OSD60-0_v9 (Autodesk Fusion 360 design; units mm, degrees)
Autodesk Fusion 360 part; units mm, degrees
sketch "Sketch1" plane through (0, 0, 0) normal (0, 0, 1) x (1, 0, 0)
  line L0 (6.985, 0.6858) -> (6.985, 4.1021)
  line L1 (6.223, 4.6101) -> (0, 4.6101)
  line L2 (0, 4.6101) -> (0, 0)
  line L3 (0, 0) -> (7.6581, 0)
  line L4 (7.6581, 0) -> (7.6581, 0.6858)
  line L5 (7.6581, 0.6858) -> (0, 0.6858)
  line L6 (0, 0.6858) -> (0, 0)
  line L7 (6.985, 4.1021) -> (6.223, 4.6101)
  point P0 (6.985, 4.6101)
  dimension "d2" = 6.985
  dimension "d3" = 7.6581
  dimension "d4" = 4.6101
  dimension "d5" = 0.6858
  dimension "d6" = 0.508
  dimension "d7" = 0.762
  constraint vertical L0
  constraint horizontal L1
  constraint vertical L2
  constraint coincident L2.end L3.start
  constraint horizontal L3
  constraint vertical L4
  constraint horizontal L5
  constraint vertical L6
  constraint coincident L0.start L5
  constraint coincident P0 L0
  constraint coincident P0 L1
  measures "d2" distance of P0 L1.end
  measures "d3" distance of L2.end L3.end
  measures "d4" distance of L2.end L1.end
  measures "d5" distance of L3.end L4.end
  measures "d6" distance of P0 L0.end
  measures "d7" distance of P0 L1.start
revolve "Revolve1" add sketch "Sketch1" angle 360 about axis through (0, 4.6101, 0) along (0, -1, 0) makes body 1
sketch "Sketch2" plane through (0, 4.6101, 0) normal (0, 1, 0) x (-1, 0, 0)
  circle A0 centre (0, 0) radius 6.223
  circle A1 centre (0, 0) radius 6.0262
  dimension "d9" = 12.0523
  constraint coincident A0.centre A1.centre
  measures "d9" diameter of A1
extrude "Extrude1" cut sketch "Sketch2" against normal blind 0.127 contours A1 bodies 1
sketch "Sketch3" plane through (0, 0, 0) normal (0, -1, 0) x (1, 0, 0)
  circle A0 centre (0, 0) radius 7.6581
  circle A1 centre (0, 0) radius 5.08 construction
  circle A2 centre (0, -5.08) radius 0.2286
  circle A3 centre (5.08, 0) radius 0.2286
  circle A4 centre (-5.08, 0) radius 0.2286
  line L0 (5.4151, 5.4151) -> (0, 0) construction
  line L1 (5.7203, 5.0917) -> (6.1872, 5.5586)
  line L2 (6.1872, 5.5586) -> (5.5586, 6.1872)
  line L3 (5.5586, 6.1872) -> (5.0917, 5.7203)
  line L4 (5.4151, 5.4151) -> (5.8729, 5.8729) construction
  line L5 (5.08, 0) -> (0, 0) construction
  line L6 (0, 0) -> (-5.08, 0) construction
  line L7 (0, 0) -> (0, -5.08) construction
  point P0 (0, -5.08)
  dimension "d12" = 10.16
  dimension "d13" = 0.4572
  dimension "d18" = 0.889
  dimension "d19" = 0.6604
  dimension "d23" = 45
  constraint coincident A0.centre A1.centre
  constraint coincident A1 P0
  constraint coincident A1 A3.centre
  constraint coincident A1 A4.centre
  constraint equal A2 A4
  constraint equal A2 A3
  constraint coincident A0 L0.start
  constraint coincident A0 L1.start
  constraint perpendicular L1 L2
  constraint coincident A0 L3.end
  constraint perpendicular L2 L3
  constraint parallel L0 L1
  constraint midpoint L2 L4.end
  constraint parallel L0 L4
  constraint coincident P0 A2.centre
  constraint perpendicular L5 L7
  constraint coincident A3.centre L5.start
  constraint coincident A4.centre L6.end
  constraint vertical L7
  constraint horizontal L6
  measures "d12" diameter of A1
  measures "d13" diameter of A2
  measures "d18" distance of L1.end L2.end
  measures "d19" distance of L1.start L1.end
  measures "d23" angle of L0 L5
extrude "Extrude2" add sketch "Sketch3" along normal blind 13.335 contours A2 | A3 | A4 bodies 1
extrude "Extrude3" add sketch "Sketch3" against normal blind 0.4064 contours A0 L1 L2 L3 bodies 1
ref_plane "WorkPlane1" through (5.6395, 0.254, 5.6395) normal (0, 1, 0) x (-1, 0, 0)
split "Split1" by plane through (5.6395, 0.254, 5.6395) normal (0, 1, 0) bodies 1 makes body 2 at (6.9763, 1.8246, -0.3482)
equation "d2 = ( 0.55 / 2 ) * 1 in"
equation "d3 = ( 0.603 / 2 ) * 1 in"
